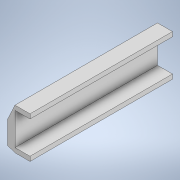
# Autodesk Inventor part: Bremslicht
Saved by Autodesk Inventor 2021 (Build 250183000, 183)
## iProperties
Created: 2021-07-20
Part Number: Bremslicht
Material: Generisch
Document SubType Name: Modeling
Designer: Lars-Ole
Density: 1 g/cm^3
Appearance: Vorgabe
Author: Lars-Ole
Autodesk Inventor part; units mm, degrees
ref_plane "YZ Plane" through (0, 0, 0) normal (1, 0, 0) x (0, 1, 0)
ref_plane "XZ Plane" through (0, 0, 0) normal (0, 1, 0) x (-1, 0, 0)
ref_plane "XY Plane" through (0, 0, 0) normal (0, 0, 1) x (1, 0, 0)
sketch "Skizze1" plane through (0, 0, 0) normal (0, 0, 1) x (1, 0, 0)
  line L0 (0, 14.473) -> (0, -7.027)
  line L1 (0, -7.027) -> (10, -7.027)
  line L2 (10, -7.027) -> (10, -10.027)
  line L3 (10, -10.027) -> (0, -10.027)
  line L4 (0, -10.027) -> (0, -7.027)
  line L5 (0, 17.473) -> (10, 17.473)
  line L6 (10, 17.473) -> (10, 14.473)
  line L7 (10, 14.473) -> (0, 14.473)
  line L8 (0, 14.473) -> (0, 17.473)
  line L9 (0, 17.473) -> (-5, 6.7505)
  line L10 (-5, 6.7505) -> (-5, -8.2495)
  line L11 (-5, -8.2495) -> (0, -10.027)
  point P0 (0, 0)
  dimension "d3" = 10
  dimension "d4" = 21.5
  dimension "d5" = 3
  dimension "d6" = 3
  dimension "d7" = 5
  dimension "d8" = 15
  dimension "d9" = 25
  constraints: 24 end point, 4 parallel, 2 horizontal, 2 perpendicular, 2 vertical, 1 point on line
  measures "d3" distance of L0.end L1.end
  measures "d4" distance between parallel lines of L1 L7
  measures "d5" distance of L5.end L6.end
  measures "d6" distance of L1.end L2.end
  measures "d7" distance between parallel lines of L0 L10
  measures "d8" distance of L10.end L9.end
  measures "d9" angle of L0 L9
extrude "Extrusion1" add sketch "Skizze1" along normal blind 95
equation "\"d6\" = d5"
